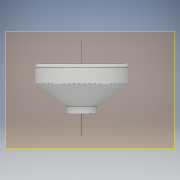
# Autodesk Inventor part: JarCone
Saved by Autodesk Inventor 2019 (Build 230136000, 136)
## iProperties
Created: 2018-12-14
Part Number: JarCone
Material: Generic
Document SubType Name: Modeling
Designer: assman
Density: 1 g/cm^3
Appearance: Default
Author: assman
Autodesk Inventor part; units mm, degrees
ref_plane "YZ Plane" through (0, 0, 0) normal (1, 0, 0) x (0, 1, 0)
ref_plane "XZ Plane" through (0, 0, 0) normal (0, 1, 0) x (-1, 0, 0)
ref_plane "Work Plane1" through (0, 0, 0) normal (0, -1, 0) x (1, 0, 0)
sketch "Sketch1" plane through (0, 0, 0) normal (0, -1, 0) x (1, 0, 0)
  circle A0 centre (0, 0) radius 52 projected
  circle A1 centre (0, 0) radius 62
  circle A2 centre (0, 0) radius 52
  dimension "d1" = 10
  constraints: 2 centre point, 2 coincident
  measures "d1" radial gap between concentric circles of A0 A1
extrude "Extrusion1" add sketch "Sketch1" against normal blind 25
sketch "Sketch3" plane through (0, 0, 0) normal (0, -1, 0) x (1, 0, 0)
  circle A0 centre (0, 0) radius 62
  circle A1 centre (0, 0) radius 50
  circle A2 centre (0, 0) radius 52 projected
  dimension "d9" = 124
  dimension "d10" = 2
  constraints: 2 centre point, 2 coincident
  measures "d9" diameter of A0
  measures "d10" radial gap between concentric circles of A2 A1
extrude "Extrusion3" add sketch "Sketch3" along normal blind 2 contours A0 | A2
sketch "Sketch4" plane through (0, -2, 0) normal (0, -1, 0) x (1, 0, 0)
  circle A0 centre (0, 0) radius 62 construction
  line L0 (-62, 0) -> (62, 0) construction
  line L1 (0, 62) -> (0, -62) construction
  constraints: 4 end point, 4 point on circle, 1 horizontal, 1 perpendicular
ref_plane "Work Plane2" through (-62, -2, 0) normal (0, 0, 1) x (1, 0, 0)
sketch "Sketch5" plane through (-62, -2, 0) normal (0, 0, 1) x (1, 0, 0)
  line L0 (0, 0) -> (124, 0) construction
  line L1 (62, 0) -> (62, -30) construction
  line L2 (62, 0) -> (62, -30) construction
  line L3 (82, -30) -> (124, 0) construction
  line L4 (62, 0) -> (62, -30) construction
  line L5 (62, 0) -> (62, -30)
  line L6 (82, -30) -> (124, 0)
  line L7 (62, 0) -> (124, 0)
  line L8 (82, -30) -> (62, -30)
  point P0 (62, 2)
  dimension "d14" = 20
  dimension "d23" = 30
  constraints: 16 end point, 5 collinear, 1 midpoint, 1 perpendicular, 1 vertical
  measures "d14" distance of L3.start L1.end
  measures "d23" distance of L1.start L1.end
revolve "Revolution1" add sketch "Sketch5" angle 360 about axis through (0, -2, 0) along (0, -1, 0)
shell "Shell1" thickness 2 removed faces 2 at (9.39, -2, -8.8667) at (-4.4202, -32, 2.9181)
fillet "Fillet2" radius 5 1 edges at (-62, 25, 0)
sketch "Sketch6" plane through (0, -32, 0) normal (0, -1, 0) x (1, 0, 0)
  circle A0 centre (0, 0) radius 20
  circle A1 centre (0, 0) radius 17.2734
  point P0 (0, 0)
  constraints: 2 centre point, 2 coincident
extrude "Extrusion4" add sketch "Sketch6" along normal blind 10
sketch "Sketch7" plane through (-62, -2, 0) normal (0, 0, 1) x (1, 0, 0)
  line L0 (116, 0) -> (8, 0) construction
  line L1 (62, 0) -> (62, -68.8676) construction
  line L2 (62, -68.8676) -> (62, 58.2557) construction
  point P0 (62, 2)
  constraints: 4 end point, 1 midpoint, 1 point on line, 1 vertical
sketch "Sketch8" plane through (0, -42, 0) normal (0, -1, 0) x (1, 0, 0)
  circle A0 centre (0, 0) radius 17.2734 construction
  circle A1 centre (0, 0) radius 20 construction
  point P0 (0, 0)
  dimension "d21" = 34.5467
  dimension "d22" = 40
  constraints: 1 centre point, 1 coincident
  measures "d21" diameter of A0
  measures "d22" diameter of A1
body "Solid1"
